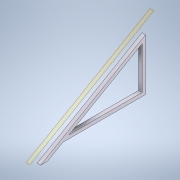
# Autodesk Inventor part: ballSupport
Saved by Autodesk Inventor 2020.2 (Build 242310000, 310)
## iProperties
Created: 2020-01-12
Part Number: ballSupport
Material: Aluminum 6061, Welded
Document SubType Name: Modeling
Designer: robst
Density: 2.7 g/cm^3
Appearance: Weld - Aluminum
Author: robst
Autodesk Inventor part; units mm, degrees
ref_plane "YZ Plane" through (0, 0, 0) normal (1, 0, 0) x (0, 1, 0)
ref_plane "XZ Plane" through (0, 0, 0) normal (0, 1, 0) x (-1, 0, 0)
ref_plane "XY Plane" through (0, 0, 0) normal (0, 0, 1) x (1, 0, 0)
sketch "Sketch1" plane through (0, 0, 0) normal (1, 0, 0) x (0, 1, 0)
  line L0 (0, 0) -> (0, -762)
  line L1 (0, -762) -> (439.9409, -762)
  line L2 (439.9409, -762) -> (0, 0)
  line L3 (25.4, -129.7892) -> (25.4, -736.6)
  line L4 (25.4, -736.6) -> (361.7607, -736.6)
  line L5 (361.7607, -736.6) -> (25.4, -129.7892)
  dimension "d0" = 762
  dimension "d5" = 30
  dimension "d6" = 1
  dimension "d7" = 25.4
  dimension "d8" = 25.4
  constraints: 12 end point, 2 perpendicular, 2 vertical
  measures "d0" distance of L0.start L0.end
  measures "d5" angle of L2 L0
  measures "d6" angle of L5 L2
  measures "d7" distance between parallel lines of L3 L0
  measures "d8" distance between parallel lines of L1 L4
extrude "Extrusion1" add sketch "Sketch1" along normal mid plane 25.4 contours L2 L1 L0 | L5 L4 L3
ref_plane "Work Plane1" through (-12.7, 65.9911, 38.1) normal (0, 0.866, 0.5) x (1, 0, 0)
sketch "Sketch3" plane through (12.7, 0, 0) normal (1, 0, 0) x (0, 0, -1)
  line L0 (0, 63.5) -> (873.76, 63.5) projected
  line L1 (204.7793, 88.9) -> (736.6, 88.9)
  line L2 (736.6, 88.9) -> (736.6, 395.9468)
  line L3 (736.6, 395.9468) -> (204.7793, 88.9)
  line L4 (762, 439.9409) -> (0, 0) projected
  line L5 (762, 0) -> (762, 439.9409) projected
  line L6 (0, 0) -> (762, 0) projected
  line L7 (50.8, 0) -> (160.7852, 63.5)
  line L8 (160.7852, 63.5) -> (762, 63.5)
  line L9 (762, 0) -> (50.8, 0)
  dimension "d14" = 25.4
  dimension "d15" = 25.4
  dimension "d21" = 25.4
  constraints: 12 end point, 4 point on line, 3 parallel, 2 collinear, 1 perpendicular
  measures "d14" distance between parallel lines of L1 L0
  measures "d15" distance between parallel lines of L2 L5
  measures "d21" distance between parallel lines of L3 L4
extrude "Extrusion4" cut sketch "Sketch3" against normal through all contours L0 L5 L6 L7 | L3 L2 L1
body "Solid1"
